Autodesk Fusion 360 part; units mm, degrees
(part 2 of 3)
sketch "dflg_DummyKey_Top_172" plane through (0, 0, -8.8) normal (0, 0, 1) x (1, 0, 0)
  line L0 (171.4, 78.4) -> (184.6, 78.4)
  line L1 (184.6, 78.4) -> (184.6, 91.6)
  line L2 (184.6, 91.6) -> (171.4, 91.6)
  line L3 (171.4, 91.6) -> (171.4, 78.4)
extrude "Extrude556" add sketch "dflg_DummyKey_Top_172" against normal blind 1.2 bodies 12
sketch "dflg_DummyKey_Top_142" plane through (0, 0, -8.8) normal (0, 0, 1) x (1, 0, 0)
  line L0 (141.4, 78.4) -> (154.6, 78.4)
  line L1 (154.6, 78.4) -> (154.6, 91.6)
  line L2 (154.6, 91.6) -> (141.4, 91.6)
  line L3 (141.4, 91.6) -> (141.4, 78.4)
extrude "Extrude557" add sketch "dflg_DummyKey_Top_142" against normal blind 1.2 bodies 13
sketch "dflg_DummyKey_Top_187" plane through (0, 0, -8.8) normal (0, 0, 1) x (1, 0, 0)
  line L0 (186.4, 78.4) -> (199.6, 78.4)
  line L1 (199.6, 78.4) -> (199.6, 91.6)
  line L2 (199.6, 91.6) -> (186.4, 91.6)
  line L3 (186.4, 91.6) -> (186.4, 78.4)
extrude "Extrude558" add sketch "dflg_DummyKey_Top_187" against normal blind 1.2 bodies 14
sketch "dflg_DummyKey_Top_202" plane through (0, 0, -8.8) normal (0, 0, 1) x (1, 0, 0)
  line L0 (201.4, 78.4) -> (214.6, 78.4)
  line L1 (214.6, 78.4) -> (214.6, 91.6)
  line L2 (214.6, 91.6) -> (201.4, 91.6)
  line L3 (201.4, 91.6) -> (201.4, 78.4)
extrude "Extrude559" add sketch "dflg_DummyKey_Top_202" against normal blind 1.2 bodies 15
sketch "dflg_DummyKey_Bot_157" plane through (0, 0, -8.8) normal (0, 0, 1) x (1, 0, 0)
  line L0 (156.4, 63.4) -> (169.6, 63.4)
  line L1 (169.6, 63.4) -> (169.6, 76.6)
  line L2 (169.6, 76.6) -> (156.4, 76.6)
  line L3 (156.4, 76.6) -> (156.4, 63.4)
extrude "Extrude560" add sketch "dflg_DummyKey_Bot_157" against normal blind 1.2 bodies 16
sketch "dflg_DummyKey_Bot_187" plane through (0, 0, -8.8) normal (0, 0, 1) x (1, 0, 0)
  line L0 (186.4, 63.4) -> (199.6, 63.4)
  line L1 (199.6, 63.4) -> (199.6, 76.6)
  line L2 (199.6, 76.6) -> (186.4, 76.6)
  line L3 (186.4, 76.6) -> (186.4, 63.4)
extrude "Extrude561" add sketch "dflg_DummyKey_Bot_187" against normal blind 1.2 bodies 17
sketch "dflg_DummyKey_Bot_142" plane through (0, 0, -8.8) normal (0, 0, 1) x (1, 0, 0)
  line L0 (141.4, 63.4) -> (154.6, 63.4)
  line L1 (154.6, 63.4) -> (154.6, 76.6)
  line L2 (154.6, 76.6) -> (141.4, 76.6)
  line L3 (141.4, 76.6) -> (141.4, 63.4)
extrude "Extrude562" add sketch "dflg_DummyKey_Bot_142" against normal blind 1.2 bodies 18
sketch "dflg_DummyKey_Bot_172" plane through (0, 0, -8.8) normal (0, 0, 1) x (1, 0, 0)
  line L0 (171.4, 63.4) -> (184.6, 63.4)
  line L1 (184.6, 63.4) -> (184.6, 76.6)
  line L2 (184.6, 76.6) -> (171.4, 76.6)
  line L3 (171.4, 76.6) -> (171.4, 63.4)
extrude "Extrude563" add sketch "dflg_DummyKey_Bot_172" against normal blind 1.2 bodies 19
sketch "dflg_DummyKey_Bot_202" plane through (0, 0, -8.8) normal (0, 0, 1) x (1, 0, 0)
  line L0 (201.4, 63.4) -> (214.6, 63.4)
  line L1 (214.6, 63.4) -> (214.6, 76.6)
  line L2 (214.6, 76.6) -> (201.4, 76.6)
  line L3 (201.4, 76.6) -> (201.4, 63.4)
extrude "Extrude564" add sketch "dflg_DummyKey_Bot_202" against normal blind 1.2 bodies 20
sketch "dflg_DummyBtn_Small_142" plane through (0, 0, -8.8) normal (0, 0, 1) x (1, 0, 0)
  line L0 (141.4, 39.4) -> (153.6, 39.4)
  line L1 (153.6, 39.4) -> (153.6, 51.6)
  line L2 (153.6, 51.6) -> (141.4, 51.6)
  line L3 (141.4, 51.6) -> (141.4, 39.4)
extrude "Extrude565" add sketch "dflg_DummyBtn_Small_142" against normal blind 1.2 bodies 21
sketch "dflg_DummyBtn_Small_155" plane through (0, 0, -8.8) normal (0, 0, 1) x (1, 0, 0)
  line L0 (154.4, 39.4) -> (166.6, 39.4)
  line L1 (166.6, 39.4) -> (166.6, 51.6)
  line L2 (166.6, 51.6) -> (154.4, 51.6)
  line L3 (154.4, 51.6) -> (154.4, 39.4)
extrude "Extrude566" add sketch "dflg_DummyBtn_Small_155" against normal blind 1.2 bodies 22
sketch "dflg_DummyBtn_Wide_139" plane through (0, 0, -8.8) normal (0, 0, 1) x (1, 0, 0)
  line L0 (138.4, 9.4) -> (165.6, 9.4)
  line L1 (165.6, 9.4) -> (165.6, 21.6)
  line L2 (165.6, 21.6) -> (138.4, 21.6)
  line L3 (138.4, 21.6) -> (138.4, 9.4)
extrude "Extrude568" add sketch "dflg_DummyBtn_Wide_139" against normal blind 1.2 bodies 23
sketch "dflg_DummyBtn_Wide_190" plane through (0, 0, -8.8) normal (0, 0, 1) x (1, 0, 0)
  line L0 (189.4, 9.4) -> (216.6, 9.4)
  line L1 (216.6, 9.4) -> (216.6, 21.6)
  line L2 (216.6, 21.6) -> (189.4, 21.6)
  line L3 (189.4, 21.6) -> (189.4, 9.4)
extrude "Extrude569" add sketch "dflg_DummyBtn_Wide_190" against normal blind 1.2 bodies 24
sketch "dflg_DummyPill_186" plane through (0, 0, -8.8) normal (0, 0, 1) x (1, 0, 0)
  line L0 (185.4, 45.4) -> (199.6, 45.4)
  line L1 (199.6, 45.4) -> (199.6, 50.6)
  line L2 (199.6, 50.6) -> (185.4, 50.6)
  line L3 (185.4, 50.6) -> (185.4, 45.4)
extrude "Extrude570" add sketch "dflg_DummyPill_186" against normal blind 1.2 bodies 25
sketch "dflg_DummyPill_202" plane through (0, 0, -8.8) normal (0, 0, 1) x (1, 0, 0)
  line L0 (201.4, 45.4) -> (215.6, 45.4)
  line L1 (215.6, 45.4) -> (215.6, 50.6)
  line L2 (215.6, 50.6) -> (201.4, 50.6)
  line L3 (201.4, 50.6) -> (201.4, 45.4)
extrude "Extrude571" add sketch "dflg_DummyPill_202" against normal blind 1.2 bodies 26
extrude "Extrude578" add 1 faces at (104.2, 86.8333, -11) along direction (0, 0, 1) blind 7 on bodies 1 bodies 1
extrude "Extrude579" add 1 faces at (102, 86.8333, -4.8) along direction (1, 0, 0) blind 1 on bodies 1 bodies 1
extrude "Extrude580" add 1 faces at (120.7617, 93, -3.3333) along direction (0, -1, 0) blind 16 on bodies 4 bodies 4
extrude "Extrude581" add 1 faces at (126.6667, 83.1667, -11) along direction (0, 0, 1) blind 8 on bodies 4 bodies 4
fillet "Fillet36" radius 2 1 edges at (130, 85, -3) on bodies 4
ref_plane "WorkPlane54" through (0, 0, -3.7) normal (0, 0, 1) x (1, 0, 0)
ref_plane "WorkPlane55" through (0, 0, -6.6) normal (0, 0, 1) x (1, 0, 0)
ref_plane "WorkPlane56" through (0, 0, -3.7) normal (0, 0, 1) x (1, 0, 0)
ref_plane "WorkPlane57" through (0, 0, -6.6) normal (0, 0, 1) x (1, 0, 0)
ref_plane "WorkPlane58" through (0, 0, -3.7) normal (0, 0, 1) x (1, 0, 0)
ref_plane "WorkPlane59" through (0, 0, -6.6) normal (0, 0, 1) x (1, 0, 0)
ref_plane "WorkPlane60" through (0, 0, -3.7) normal (0, 0, 1) x (1, 0, 0)
ref_plane "WorkPlane61" through (0, 0, -6.6) normal (0, 0, 1) x (1, 0, 0)
ref_plane "WorkPlane62" through (0, 0, -3.7) normal (0, 0, 1) x (1, 0, 0)
ref_plane "WorkPlane63" through (0, 0, -6.6) normal (0, 0, 1) x (1, 0, 0)
ref_plane "WorkPlane64" through (0, 0, -3.7) normal (0, 0, 1) x (1, 0, 0)
ref_plane "WorkPlane65" through (0, 0, -6.4) normal (0, 0, 1) x (1, 0, 0)
extrude "Extrude645" cut 1 faces at (63.1792, 74.7218, -20.4) along direction (0, 0, 1) blind 14 on bodies 1 bodies 1
extrude "Extrude646" cut 1 faces at (59.609, 74.3228, -15.9) along direction (0, 0, 1) blind 9.5 on bodies 1 bodies 1
extrude "Extrude647" add 1 faces at (96.6851, 105.8013, -16.4) along direction (0, 0, -1) blind 8 on bodies 1 bodies 1
extrude "Extrude648" add 1 faces at (14.3667, 106, -16.4) along direction (0, 0, -1) blind 8 on bodies 1 bodies 1
extrude "Extrude649" add 1 faces at (83, 113.2, -6.1333) along direction (-1, 0, 0) blind 3 on bodies 1 bodies 1
extrude "Extrude650" cut 1 faces at (14.3667, 106, -24.4) along direction (0, 0, 1) blind 3 on bodies 1 bodies 1
extrude "Extrude651" cut 1 faces at (96.6851, 105.8013, -24.4) along direction (0, 0, 1) blind 3 on bodies 1 bodies 1
extrude "Extrude652" add 1 faces at (96.6851, 105.8013, -21.4) along direction (0, 0, -1) blind 0.5 on bodies 1 bodies 1
extrude "Extrude653" add 1 faces at (14.3667, 106, -21.4) along direction (0, 0, -1) blind 0.5 on bodies 1 bodies 1
move_face "MoveFace1" by (-5, 0, 0) 1 faces at (86.3, 115.1, -5.6) on bodies 1
extrude "Extrude654" add 1 faces at (88.5, 81.5, -5.8667) along direction (-1, 0, 0) blind 23 on bodies 1 bodies 1
extrude "Extrude655" add 1 faces at (88.5, 78.6833, -5.8667) along direction (-1, 0, 0) blind 23 on bodies 1 bodies 1
extrude "Extrude656" cut 1 faces at (24.7, 98.8, -6.1333) along direction (-1, 0, 0) blind 1 on bodies 1 bodies 1
extrude "Extrude657" add 1 faces at (80, 113.2, -6.1333) along direction (-1, 0, 0) blind 2 on bodies 1 bodies 1
extrude "Extrude658" add 1 faces at (65.5, 75.3, -5.3333) along direction (1, 0, 0) blind 9 on bodies 1 bodies 1
extrude "Extrude659" add 4 faces at (65.5, 73, -4.8) (65.5, 70, -4.8) (65.5, 67, -4.8) (65.5, 64, -4.8) along direction (1, 0, 0) blind 9 on bodies 1 bodies 1
extrude "Extrude660" add 1 faces at (77.5, 75.9, -4.5333) along direction (0, -1, 0) blind 1 on bodies 1 bodies 1
extrude "Extrude661" add 1 faces at (77.5, 76, -5.6) along direction (0, 0, -1) blind 0.7 on bodies 1 bodies 1
extrude "Extrude662" add 1 faces at (77.5, 76, -6.3) along direction (0, 0, -1) blind 0.1 on bodies 1 bodies 1
extrude "Extrude663" cut 1 faces at (10.1851, 75.8013, -20.4) along direction (0, 0, 1) blind 4.5 on bodies 1 bodies 1
extrude "Extrude664" cut 1 faces at (4.8353, 75.2763, -15.9) along direction (0, 0, 1) blind 9.5 on bodies 1 bodies 1
extrude "Extrude665" cut 1 faces at (94.1792, 53.7218, -20.4) along direction (0, 0, 1) blind 4.5 on bodies 1 bodies 1
extrude "Extrude666" cut 1 faces at (88.7042, 55.1056, -15.9) along direction (0, 0, 1) blind 9.5 on bodies 1 bodies 1
extrude "Extrude667" cut 1 faces at (51.1892, 20.6651, -20.4) along direction (0, 0, 1) blind 4.5 on bodies 1 bodies 1
extrude "Extrude668" cut 1 faces at (48.3181, 21.1557, -15.9) along direction (0, 0, 1) blind 9.5 on bodies 1 bodies 1
extrude "Extrude669" cut 1 faces at (12.1792, 24.7218, -20.4) along direction (0, 0, 1) blind 4.5 on bodies 1 bodies 1
extrude "Extrude670" cut 1 faces at (8.7033, 26.2999, -15.9) along direction (0, 0, 1) blind 9.5 on bodies 1 bodies 1
ref_plane "WorkPlane66" through (52.5, 80.0825, -6.4) normal (0, 0, -1) x (-1, 0, 0)
sketch "Sketch596" plane through (0, 0, -6.4) normal (0, 0, -1) x (-1, 0, 0)
  line L0 (-2.4, 78.2245) -> (-8.4, 78.2245)
  line L1 (-8.4, 78.2245) -> (-8.4, 16.2245)
  line L2 (-8.4, 16.2245) -> (-2.4, 16.2245)
  line L3 (-2.4, 16.2245) -> (-2.4, 78.2245)
  line L4 (-2.4, 6) -> (-2.4, 138.2533)
  dimension "d1957" = 6
  dimension "d1958" = 62
  constraint horizontal L0
  constraint vertical L1
  constraint horizontal L2
  constraint vertical L3
  constraint coincident L0.start L4
  measures "d1957" distance of L0.start L0.end
  measures "d1958" distance of L0.start L2.end
extrude "Extrude671" add sketch "Sketch596" along normal blind 3 bodies 1
extrude "Extrude672" cut 1 faces at (4.4, 36.8912, -9.4) along direction (0, 0, 1) blind 1 on bodies 1 bodies 1
sketch "Sketch597" plane through (0, 0, -8.4) normal (0, 0, -1) x (1, 0, 0)
  line L0 (8.4, -16.2245) -> (2.4, -16.2245)
  line L1 (2.4, -16.2245) -> (2.4, -78.2245)
  line L2 (2.4, -78.2245) -> (8.4, -78.2245)
  line L3 (8.4, -78.2245) -> (8.4, -16.2245)
  circle A0 centre (5, -73) radius 1.6
  circle A1 centre (5, -51) radius 1.6
  circle A2 centre (5, -29) radius 1.6
  circle A3 centre (68, -70) radius 1.6
  circle A4 centre (53, -29) radius 1.6
  circle A5 centre (69, -73) radius 1.6
  circle A6 centre (69, -73) radius 1.6
  circle A7 centre (69.5, -72.5) radius 1.6
  dimension "d1963" = 3.2
  dimension "d1966" = 0
  dimension "d1967" = 44
  dimension "d1980" = 3.2
  dimension "d2000" = 3.2
  dimension "d2003" = 3.2
  dimension "d2016" = 3.2
  constraint concentric A5 A6
  measures "d1963" diameter of A0
  measures "d1980" diameter of A3
  measures "d2000" diameter of A5
  measures "d2003" diameter of A6
  measures "d2016" diameter of A7
extrude "Extrude673" add sketch "Sketch597" along normal blind 1 contours L0 L1 L2 L3 bodies 1
extrude "Extrude674" cut 3 faces at (4.8052, 72.5035, -8.4) (5.391, 51.3628, -8.4) (4.7333, 28.5381, -8.4) along direction (0, 0, 1) blind 2.5 on bodies 1 bodies 1
extrude "Extrude675" add 4 faces at (74.5, 73, -4.8) (74.5, 70, -4.8) (74.5, 67, -4.8) (74.5, 64, -4.8) along direction (1, 0, 0) blind 5 on bodies 1 bodies 1
extrude "Extrude676" cut 4 faces at (83.5, 63.5, -4.8) (83.5, 66.5, -4.8) (83.5, 69.5, -4.8) (83.5, 72.5, -4.8) along direction (1, 0, 0) blind 11 on bodies 1 bodies 1
sketch "Sketch598" plane through (0, 0, -6.4) normal (0, 0, -1) x (1, 0, 0)
  line L0 (8.4, -78.2245) -> (2.4, -78.2245)
  line L1 (2.4, -78.2245) -> (2.4, -138.2533)
  arc A0 (53.3792, -143.3184) -> (2.4, -138.2533) centre (11.7114, -303.6168) ccw
  arc A1 (102.6, -157.7649) -> (53.3792, -143.3184) centre (-358, -1636) ccw
  line L2 (102.6, -157.7649) -> (102.6, -6)
  arc A2 (102.6, -6) -> (99, -2.4) centre (99, -6) ccw
  line L3 (99, -2.4) -> (6, -2.4)
  arc A3 (6, -2.4) -> (2.4, -6) centre (6, -6) ccw
  line L4 (2.4, -6) -> (2.4, -16.2245)
  line L5 (2.4, -16.2245) -> (8.4, -16.2245)
  line L6 (8.4, -16.2245) -> (8.4, -78.2245)
  circle A4 centre (40, -69) radius 7.2
  circle A5 centre (30, -32.5) radius 7.2
  circle A6 centre (93.5, -106) radius 4
  line L7 (76.65, -139.05) -> (88.65, -139.05)
  line L8 (88.65, -139.05) -> (88.65, -142.05)
  line L9 (88.65, -142.05) -> (76.65, -142.05)
  line L10 (76.65, -142.05) -> (76.65, -139.05)
  circle A7 centre (93, -11.5) radius 4.2
  circle A8 centre (11.5, -11.5) radius 4.2
  line L11 (59, -25.8) -> (71.3, -25.8)
  line L12 (71.3, -25.8) -> (71.3, -13.5)
  line L13 (71.3, -13.5) -> (83.7, -13.5)
  line L14 (83.7, -13.5) -> (83.7, -25.8)
  line L15 (83.7, -25.8) -> (96, -25.8)
  line L16 (96, -25.8) -> (96, -38.2)
  line L17 (96, -38.2) -> (83.7, -38.2)
  line L18 (83.7, -38.2) -> (83.7, -50.5)
  line L19 (83.7, -50.5) -> (71.3, -50.5)
  line L20 (71.3, -50.5) -> (71.3, -38.2)
  line L21 (71.3, -38.2) -> (59, -38.2)
  line L22 (59, -38.2) -> (59, -25.8)
  line L23 (61.8432, -78.55) -> (88.65, -78.55)
  line L24 (88.65, -78.55) -> (88.65, -130.45)
  line L25 (88.65, -130.45) -> (85.65, -130.45)
  line L26 (85.65, -130.45) -> (85.65, -81.55)
  line L27 (85.65, -81.55) -> (18.95, -81.55)
  line L28 (18.95, -81.55) -> (18.95, -130.45)
  line L29 (18.95, -130.45) -> (15.95, -130.45)
  line L30 (15.95, -130.45) -> (15.95, -78.55)
  line L31 (15.95, -78.55) -> (58.1568, -78.55)
  arc A9 (58.1568, -78.55) -> (61.8432, -78.55) centre (60, -75) ccw
  line L32 (19.5567, -75.9) -> (15.4433, -75.9)
  arc A10 (19.5567, -75.9) -> (15.4433, -75.9) centre (17.5, -69) ccw
  line L33 (49.5, -54) -> (64.5, -54)
  line L34 (64.5, -54) -> (64.5, -58)
  line L35 (64.5, -58) -> (49.5, -58)
  line L36 (49.5, -58) -> (49.5, -54)
  line L37 (30.5, -54) -> (45.5, -54)
  line L38 (45.5, -54) -> (45.5, -58)
  line L39 (45.5, -58) -> (30.5, -58)
  line L40 (30.5, -58) -> (30.5, -54)
  circle A11 centre (93, -80) radius 4.2
  circle A12 centre (11.5, -85) radius 4.2
  circle A13 centre (93, -120) radius 4.2
  circle A14 centre (11.5, -106) radius 4
  line L41 (78, -127.6) -> (23.7, -127.6)
  line L42 (23.7, -127.6) -> (23.7, -84.4)
  line L43 (23.7, -84.4) -> (78, -84.4)
  line L44 (78, -84.4) -> (78, -127.6)
  line L45 (94.5, -73.5) -> (79.5, -73.5)
  line L46 (79.5, -73.5) -> (79.5, -72)
  line L47 (79.5, -72) -> (94.5, -72)
  line L48 (94.5, -72) -> (94.5, -73.5)
  line L49 (94.5, -67.5) -> (79.5, -67.5)
  line L50 (79.5, -67.5) -> (79.5, -66)
  line L51 (79.5, -66) -> (94.5, -66)
  line L52 (94.5, -66) -> (94.5, -67.5)
  line L53 (94.5, -64.5) -> (79.5, -64.5)
  line L54 (79.5, -64.5) -> (79.5, -63)
  line L55 (79.5, -63) -> (94.5, -63)
  line L56 (94.5, -63) -> (94.5, -64.5)
  line L57 (94.5, -70.5) -> (79.5, -70.5)
  line L58 (79.5, -70.5) -> (79.5, -69)
  line L59 (79.5, -69) -> (94.5, -69)
  line L60 (94.5, -69) -> (94.5, -70.5)
  line L61 (83.2556, -76.4857) -> (65.2556, -76.4857)
  line L62 (65.2556, -76.4857) -> (65.2556, -52.4857)
  line L63 (65.2556, -52.4857) -> (83.2556, -52.4857)
  line L64 (83.2556, -52.4857) -> (83.2556, -76.4857)
  line L65 (58, -45) -> (49, -45)
  line L66 (49, -45) -> (49, -17)
  line L67 (49, -17) -> (58, -17)
  line L68 (58, -17) -> (58, -45)
  dimension "d1976" = 24
  dimension "d1977" = 18
  constraint horizontal L61
  constraint vertical L62
  constraint horizontal L63
  constraint vertical L64
  constraint horizontal L65
  constraint vertical L66
  constraint horizontal L67
  constraint vertical L68
  measures "d1976" distance of L61.start L63.end
  measures "d1977" distance of L61.start L61.end
extrude "Extrude678" add sketch "Sketch598" along normal blind 3 contours L65 L66 L67 L68 bodies 1
extrude "Extrude679" cut sketch "Sketch597" against normal blind 3.5 contours A3 A7 | A3 A5 A6 A7 | A3 A5 A6 picked at (68.8187, -71.1587) bodies 1
sketch "Sketch599" plane through (0, 0, -9.4) normal (0, 0, -1) x (1, 0, 0)
  line L0 (58, -17) -> (49, -17)
  line L1 (49, -17) -> (49, -45)
  line L2 (49, -45) -> (58, -45)
  line L3 (58, -45) -> (58, -17)
  circle A0 centre (53, -29) radius 1.6
  circle A1 centre (54, -30) radius 1.6
  dimension "d1986" = 3.2
  dimension "d2007" = 3.2
  measures "d1986" diameter of A0
  measures "d2007" diameter of A1
extrude "Extrude680" cut sketch "Sketch599" against normal blind 3.5 contours A0 A1 | A0 A1 picked at (53.3119, -29.2702) picked at (52.5374, -28.5374) bodies 1
extrude "Extrude681" add 4 faces at (79.5, 73, -4.8) (79.5, 70, -4.8) (79.5, 67, -4.8) (79.5, 64, -4.8) along direction (1, 0, 0) blind 6.5 on bodies 1 bodies 1
extrude "Extrude682" cut 4 faces at (94.5, 72.5, -4.8) (94.5, 69.5, -4.8) (94.5, 66.5, -4.8) (94.5, 63.5, -4.8) along direction (1, 0, 0) blind 5 on bodies 1 bodies 1
extrude "Extrude683" add sketch "Sketch598" along normal blind 3 contours L45 L46 L47 L49 L50 L51 L53 L54 L55 L57 L58 L59 L61 L62 L63 L64 | L45 L46 L47 L64 | L57 L58 L59 L64 | L49 L50 L51 L64 | L53 L54 L55 L64 bodies 1
sketch "Sketch600" plane through (0, 0, -9.4) normal (0, 0, -1) x (1, 0, 0)
  line L0 (83.2556, -52.4857) -> (65.2556, -52.4857)
  line L1 (65.2556, -52.4857) -> (65.2556, -76.4857)
  line L2 (65.2556, -76.4857) -> (83.2556, -76.4857)
  line L3 (83.2556, -76.4857) -> (83.2556, -52.4857)
  circle A0 centre (77, -59) radius 1.6
  dimension "d2028" = 3.2
  measures "d2028" diameter of A0
extrude "Extrude685" add sketch "Sketch597" along normal blind 1 contours A3 A7 | A3 A5 A6 A7 picked at (68.8187, -71.1587) bodies 1
extrude "Extrude687" add sketch "Sketch599" along normal blind 1 separate body contours A0 A1 | A0 A1 picked at (53.3119, -29.2702) picked at (52.5374, -28.5374) makes body 27
extrude "Extrude688" cut 1 faces at (53.4404, 28.6598, -10.4) along direction (0, 0, 1) blind 1 on bodies 27 bodies 27
extrude "Extrude689" add sketch "Sketch597" along normal blind 1 contours A4 bodies 1 27
extrude "Extrude690" cut sketch "Sketch599" against normal blind 3.5 contours A0 A1 | A0 A1 picked at (53.3119, -29.2702) picked at (54.988, -30.5494) bodies 1
extrude "Extrude691" add sketch "Sketch597" along normal blind 1 separate body contours A5 A6 A7 makes body 28
sketch "Sketch602" plane through (0, 0, -9.4) normal (0, 0, -1) x (1, 0, 0)
  circle A0 centre (69.5, -72.5) radius 1.6
  dimension "d2019" = 3.2
  measures "d2019" diameter of A0
extrude "Extrude692" cut sketch "Sketch602" against normal blind 3.5 bodies 1
extrude "Extrude693" add sketch "Sketch600" against normal blind 5 contours L0 L1 L2 L3 | A0 bodies 1 28
extrude "Extrude694" cut sketch "Sketch602" against normal blind 3.5 bodies 1
sketch "Sketch603" plane through (0, 0, -6.4) normal (0, 0, -1) x (1, 0, 0)
sketch "Sketch604" plane through (0, 0, -6.4) normal (0, 0, -1) x (1, 0, 0)
  line L0 (49, -17) -> (49, -6)
  line L1 (49, -6) -> (69, -6)
  line L2 (69, -6) -> (69, -17)
  line L3 (69, -17) -> (49, -17)
  line L4 (58, -24) -> (68, -24)
  line L5 (68, -24) -> (68, -17)
  line L6 (68, -17) -> (58, -17)
  line L7 (58, -17) -> (58, -24)
  line L8 (58, -40) -> (69, -40)
  line L9 (69, -40) -> (69, -51)
  line L10 (69, -51) -> (58, -51)
  line L11 (58, -51) -> (58, -40)
  line L12 (86, -16) -> (86, -25)
  line L13 (86, -25) -> (101.3332, -25)
  line L14 (101.3332, -25) -> (101.3332, -16)
  line L15 (101.3332, -16) -> (86, -16)
  line L16 (97, -25) -> (97, -57)
  line L17 (97, -57) -> (102, -57)
  line L18 (102, -57) -> (102, -25)
  line L19 (102, -25) -> (97, -25)
  line L20 (97, -41) -> (86, -41)
  line L21 (86, -41) -> (86, -57)
  line L22 (86, -57) -> (97, -57)
  line L23 (97, -57) -> (97, -41)
  constraint perpendicular L0 L1
  constraint parallel L0 L2
  constraint parallel L1 L3
  constraint vertical L0
  constraint perpendicular L4 L5
  constraint parallel L4 L6
  constraint parallel L5 L7
  constraint perpendicular L2 L4
  constraint perpendicular L8 L9
  constraint parallel L8 L10
  constraint parallel L9 L11
  constraint horizontal L8
  constraint perpendicular L12 L13
  constraint parallel L12 L14
  constraint parallel L13 L15
  constraint perpendicular L10 L12
  constraint perpendicular L16 L17
  constraint parallel L16 L18
  constraint parallel L17 L19
  constraint perpendicular L13 L16
  constraint coincident L13 L16.start
  constraint perpendicular L20 L21
  constraint parallel L20 L22
  constraint parallel L21 L23
  constraint perpendicular L16 L20
  constraint midpoint L16 L20.start
extrude "Extrude695" add sketch "Sketch604" along normal blind 3 bodies 1
sketch "Sketch605" plane through (0, 0, -9.4) normal (0, 0, -1) x (1, 0, 0)
  circle A0 centre (54, -30) radius 1.6
  line L0 (49, -6) -> (49, -45)
  line L1 (49, -45) -> (58, -45)
  line L2 (58, -45) -> (58, -51)
  line L3 (58, -51) -> (69, -51)
  line L4 (69, -51) -> (69, -40)
  line L5 (69, -40) -> (58, -40)
  line L6 (58, -40) -> (58, -24)
  line L7 (58, -24) -> (68, -24)
  line L8 (68, -24) -> (68, -17)
  line L9 (68, -17) -> (69, -17)
  line L10 (69, -17) -> (69, -6)
  line L11 (69, -6) -> (49, -6)
  circle A1 centre (63, -11) radius 1.6
  dimension "d2029" = 3.2
  measures "d2029" diameter of A1
sketch "Sketch606" plane through (0, 0, -9.4) normal (0, 0, -1) x (1, 0, 0)
  line L0 (86, -57) -> (102, -57)
  line L1 (102, -57) -> (102, -25)
  line L2 (102, -25) -> (101.3332, -25)
  line L3 (101.3332, -25) -> (101.3332, -16)
  line L4 (101.3332, -16) -> (86, -16)
  line L5 (86, -16) -> (86, -25)
  line L6 (86, -25) -> (97, -25)
  line L7 (97, -25) -> (97, -41)
  line L8 (97, -41) -> (86, -41)
  line L9 (86, -41) -> (86, -57)
  circle A0 centre (95, -47) radius 1.6
  circle A1 centre (92, -21) radius 1.6
  dimension "d2030" = 3.2
  dimension "d2031" = 3.2
  measures "d2030" diameter of A0
  measures "d2031" diameter of A1
extrude "Extrude696" cut sketch "Sketch606" against normal blind 3.5 contours A0 | A1 bodies 1
extrude "Extrude697" cut sketch "Sketch605" against normal blind 3.5 contours A1 bodies 1
extrude "Extrude698" cut sketch "Sketch600" against normal blind 3.5 contours A0 bodies 1
sketch "Sketch607" plane through (0, 0, -9.4) normal (0, 0, -1) x (1, 0, 0)
  circle A0 centre (63, -11) radius 1.6
  circle A1 centre (54, -30) radius 1.6
  line L0 (49, -6) -> (49, -45)
  line L1 (49, -45) -> (58, -45)
  line L2 (58, -45) -> (58, -51)
  line L3 (58, -51) -> (69, -51)
  line L4 (69, -51) -> (69, -40)
  line L5 (69, -40) -> (58, -40)
  line L6 (58, -40) -> (58, -24)
  line L7 (58, -24) -> (68, -24)
  line L8 (68, -24) -> (68, -17)
  line L9 (68, -17) -> (69, -17)
  line L10 (69, -17) -> (69, -6)
  line L11 (69, -6) -> (49, -6)
  circle A2 centre (65, -45) radius 1.75
  dimension "d2038" = 3.5
  measures "d2038" diameter of A2
extrude "Extrude699" cut sketch "Sketch607" against normal blind 3.5 contours A2 bodies 1
extrude "Extrude677" add sketch "Sketch598" along normal blind 3 contours L45 L46 L47 L49 L50 L51 L53 L54 L55 L57 L58 L59 L61 L62 L63 L64 | L45 L46 L47 L64 | L57 L58 L59 L64 | L49 L50 L51 L64 | L53 L54 L55 L64 bodies 1
ref_plane "WorkPlane67" through (0, 155, 0) normal (0, 1, 0) x (0, 0, 1)
sketch "Sketch614" plane through (0, 0, -8) normal (0, 0, -1) x (1, 0, 0)
  line L0 (15.95, -142.05) -> (15.95, -141.849)
  arc A0 (15.95, -141.849) -> (14.1534, -167.6) centre (19, -155) ccw
  line L1 (14.1534, -167.6) -> (23.8466, -167.6)
  arc A1 (23.8466, -167.6) -> (22.8141, -142.05) centre (19, -155) ccw
  line L2 (22.8141, -142.05) -> (15.95, -142.05)
  circle A2 centre (11.5, -156) radius 4.2
sketch "Sketch615" plane through (0, 0, 5.8) normal (0, 0, 1) x (-1, 0, 0)
  circle A0 centre (-19, -155) radius 13.5
  circle A1 centre (-19, -155) radius 1.5
  dimension "d2062" = 3
  constraint concentric A0 A1
  measures "d2062" diameter of A1
extrude "Extrude703" cut sketch "Sketch615" against normal blind 30 contours A1 bodies 1
extrude "Extrude704" cut sketch "Sketch602" against normal blind 3.5 bodies 1
sketch "Sketch616" plane through (0, 0, -9.4) normal (0, 0, -1) x (1, 0, 0)
  circle A0 centre (69.5, -72.5) radius 1.6
  line L0 (83.2556, -52.4857) -> (65.2556, -52.4857)
  line L1 (65.2556, -52.4857) -> (65.2556, -76.4857)
  line L2 (65.2556, -76.4857) -> (83.2556, -76.4857)
  line L3 (83.2556, -76.4857) -> (83.2556, -52.4857)
  circle A1 centre (77, -59) radius 1.6
  dimension "d2067" = 3.2
  measures "d2067" diameter of A1
extrude "Extrude705" cut sketch "Sketch616" against normal blind 3.5 contours A1 bodies 1
extrude "Extrude706" add sketch "Sketch599" against normal blind 3.5 contours A0 A1 picked at (52.5374, -28.5374) bodies 1
extrude "Extrude707" cut 1 faces at (40.5, 58, -4.8) along direction (0, 1, 0) blind 0.5 on bodies 1 bodies 1
extrude "Extrude708" cut 1 faces at (59.5, 58, -4.8) along direction (0, 1, 0) blind 0.5 on bodies 1 bodies 1
extrude "Extrude709" cut 1 faces at (54.5, 54, -4.8) along direction (0, -1, 0) blind 0.5 on bodies 1 bodies 1
extrude "Extrude710" cut 1 faces at (35.5, 54, -4.8) along direction (0, -1, 0) blind 0.5 on bodies 1 bodies 1
sketch "Sketch617" plane through (0, 0, -8) normal (0, 0, -1) x (1, 0, 0)
  circle A0 centre (19, -155) radius 1.5
  dimension "d2080" = 3
  measures "d2080" diameter of A0
extrude "Extrude711" add sketch "Sketch617" against normal blind 13.4 bodies 1
sketch "Sketch618" plane through (0, 0, 5.8) normal (0, 0, 1) x (-1, 0, 0)
  circle A0 centre (-19, -155) radius 1.5
  circle A1 centre (-19, -155) radius 13.5
  line L0 (-11.5, -150) -> (-26.5, -150)
  line L1 (-26.5, -150) -> (-26.5, -160)
  line L2 (-26.5, -160) -> (-11.5, -160)
  line L3 (-11.5, -160) -> (-11.5, -150)
  line L4 (-11.5, -150) -> (-26.5, -160) construction
  line L5 (-26.5, -150) -> (-11.5, -160) construction
  point P0 (-19, -155)
  dimension "d2083" = 15
  dimension "d2084" = 10
  constraint horizontal L0
  constraint perpendicular L0 L1
  constraint parallel L0 L2
  constraint parallel L1 L3
  constraint coincident L4 P0
  constraint coincident L5 P0
  constraint coincident P0 A0.centre
  measures "d2083" distance of L1.end L2.end
  measures "d2084" distance of L0.end L1.end
extrude "Extrude712" cut sketch "Sketch618" against normal blind 0.5 contours L0 L1 L2 L3 bodies 1
extrude "Extrude713" cut 1 faces at (19.25, 155.433, 5.4) along direction (0, 0, -1) blind 0.2 on bodies 1 bodies 1
extrude "Extrude714" add 1 faces at (19.25, 155.433, 5.2) along direction (0, 0, 1) blind 0.1 on bodies 1 bodies 1
sketch "Sketch619" plane through (0, 0, 5.8) normal (0, 0, 1) x (-1, 0, 0)
  line L0 (-26.5, -150) -> (-11.5, -150)
  line L1 (-11.5, -150) -> (-11.5, -160)
  line L2 (-11.5, -160) -> (-26.5, -160)
  line L3 (-26.5, -160) -> (-26.5, -150)
  circle A0 centre (-19, -155) radius 13.5
  line L4 (-27.5, -160) -> (-29, -160)
  line L5 (-29, -160) -> (-29, -150)
  line L6 (-29, -150) -> (-27.5, -150)
  line L7 (-27.5, -150) -> (-27.5, -160)
  constraint horizontal L4
  constraint vertical L5
  constraint horizontal L6
  constraint vertical L7
extrude "Extrude715" cut sketch "Sketch619" against normal blind 23 contours L4 L5 L6 L7 bodies 1
sketch "Sketch620" plane through (0, 0, -6.4) normal (0, 0, -1) x (1, 0, 0)
extrude "Extrude716" cut 1 faces at (54.5, 53.5, -4.8) along direction (0, -1, 0) blind 2.4 on bodies 1 bodies 1
extrude "Extrude717" cut 1 faces at (35.5, 53.5, -4.8) along direction (0, -1, 0) blind 2.4 on bodies 1 bodies 1
extrude "Extrude718" cut 4 faces at (61.891, 105.5419, -34) (9.891, 100.4419, -34) (9.891, 72.4419, -34) (60.591, 57.2419, -34) along direction (0, 0, -1) blind 6 on bodies 3 bodies 3
extrude "Extrude719" cut 1 faces at (40.5, 58.5, -4.8) along direction (0, 1, 0) blind 1.2 on bodies 1 bodies 1
extrude "Extrude720" cut 1 faces at (59.5, 58.5, -4.8) along direction (0, 1, 0) blind 1.2 on bodies 1 bodies 1
extrude "Extrude721" cut 1 faces at (8.1408, 84.1822, -44) along direction (0, 0, 1) blind 6 on bodies 1 bodies 1
extrude "Extrude722" cut 1 faces at (8.1408, 84.1822, -38) along direction (0, 0, 1) blind 0.5 on bodies 1 bodies 1
extrude "Extrude723" cut 1 faces at (8.3797, 84.2559, -37.5) along direction (0, 0, 1) blind 31 on bodies 1 bodies 1
extrude "Extrude724" cut 1 faces at (11.4689, 84.1151, -32.4) along direction (0, 0, 1) blind 26 on bodies 1 bodies 1
sketch "delboss_66_1007" plane through (0, 0, 0) normal (0, 0, 1) x (1, 0, 0)
  circle A0 centre (6.6, 100.7) radius 5.5
extrude "Extrude729" cut sketch "delboss_66_1007" along normal blind 4.02 from surface at -44.01 bodies 3
sketch "delboss_586_1058" plane through (0, 0, 0) normal (0, 0, 1) x (1, 0, 0)
  circle A0 centre (58.6, 105.8) radius 5.5
extrude "Extrude730" cut sketch "delboss_586_1058" along normal blind 4.02 from surface at -44.01 bodies 3
sketch "delboss_573_575" plane through (0, 0, 0) normal (0, 0, 1) x (1, 0, 0)
  circle A0 centre (57.3, 57.5) radius 5.5
extrude "Extrude731" cut sketch "delboss_573_575" along normal blind 4.02 from surface at -44.01 bodies 3
sketch "delboss_66_727" plane through (0, 0, 0) normal (0, 0, 1) x (1, 0, 0)
  circle A0 centre (6.6, 72.7) radius 5.5
extrude "Extrude732" cut sketch "delboss_66_727" along normal blind 4.02 from surface at -44.01 bodies 3
sketch "nboss_537_420" plane through (0, 0, 0) normal (0, 0, 1) x (1, 0, 0)
  circle A0 centre (53.7, 42) radius 4
extrude "Extrude733" add sketch "nboss_537_420" along normal blind 4 from surface at -44 bodies 3
sketch "nbore_537_420" plane through (0, 0, 0) normal (0, 0, 1) x (1, 0, 0)
  circle A0 centre (53.7, 42) radius 2
extrude "Extrude734" cut sketch "nbore_537_420" against normal blind 3 from surface at -40 bodies 3
sketch "nboss_588_940" plane through (0, 0, 0) normal (0, 0, 1) x (1, 0, 0)
  circle A0 centre (58.8, 94) radius 4
extrude "Extrude735" add sketch "nboss_588_940" along normal blind 4 from surface at -44 bodies 3
sketch "nbore_588_940" plane through (0, 0, 0) normal (0, 0, 1) x (1, 0, 0)
  circle A0 centre (58.8, 94) radius 2
extrude "Extrude736" cut sketch "nbore_588_940" against normal blind 3 from surface at -40 bodies 3
sketch "nboss_105_927" plane through (0, 0, 0) normal (0, 0, 1) x (1, 0, 0)
  circle A0 centre (10.5, 92.7) radius 4
extrude "Extrude737" add sketch "nboss_105_927" along normal blind 4 from surface at -44 bodies 3
sketch "nbore_105_927" plane through (0, 0, 0) normal (0, 0, 1) x (1, 0, 0)
  circle A0 centre (10.5, 92.7) radius 2
extrude "Extrude738" cut sketch "nbore_105_927" against normal blind 3 from surface at -40 bodies 3
sketch "nboss_257_420" plane through (0, 0, 0) normal (0, 0, 1) x (1, 0, 0)
  circle A0 centre (25.7, 42) radius 4
extrude "Extrude739" add sketch "nboss_257_420" along normal blind 4 from surface at -44 bodies 3
sketch "nbore_257_420" plane through (0, 0, 0) normal (0, 0, 1) x (1, 0, 0)
  circle A0 centre (25.7, 42) radius 2
extrude "Extrude740" cut sketch "nbore_257_420" against normal blind 3 from surface at -40 bodies 3
sketch "unoq_rot" plane through (0, 0, 0) normal (0, 0, 1) x (1, 0, 0)
  line L0 (8, 39.4) -> (61.3, 39.4)
  line L1 (61.3, 39.4) -> (61.3, 108)
  line L2 (61.3, 108) -> (8, 108)
  line L3 (8, 108) -> (8, 39.4)
extrude "Extrude741" add sketch "unoq_rot" along normal blind 9.6 from surface at -34 separate body makes body 29
sketch "usbc_rot" plane through (0, 0, 0) normal (0, 0, 1) x (1, 0, 0)
  line L0 (12, 108) -> (21, 108)
  line L1 (21, 108) -> (21, 111.4)
  line L2 (21, 111.4) -> (12, 111.4)
  line L3 (12, 111.4) -> (12, 108)
extrude "Extrude742" add sketch "usbc_rot" along normal blind 3.2 from surface at -34 separate body makes body 30
sketch "mount_base" plane through (0, 0, 0) normal (0, 0, 1) x (1, 0, 0)
  line L0 (127, 17) -> (201.6, 17)
  line L1 (201.6, 17) -> (201.6, 76.3)
  line L2 (201.6, 76.3) -> (127, 76.3)
  line L3 (127, 76.3) -> (127, 17)
extrude "Extrude743" add sketch "mount_base" along normal blind 3 separate body makes body 31
sketch "mstand_26_457" plane through (0, 0, 0) normal (0, 0, 1) x (1, 0, 0)
  circle A0 centre (132.6, 65.7) radius 3.5
extrude "Extrude744" add sketch "mstand_26_457" along normal blind 6 from surface at 3 bodies 31
sketch "mpilot_26_457" plane through (0, 0, 0) normal (0, 0, 1) x (1, 0, 0)
  circle A0 centre (132.6, 65.7) radius 1.35
extrude "Extrude745" cut sketch "mpilot_26_457" against normal blind 7 from surface at 9 bodies 31
sketch "mstand_546_508" plane through (0, 0, 0) normal (0, 0, 1) x (1, 0, 0)
  circle A0 centre (184.6, 70.8) radius 3.5
extrude "Extrude746" add sketch "mstand_546_508" along normal blind 6 from surface at 3 bodies 31
sketch "mpilot_546_508" plane through (0, 0, 0) normal (0, 0, 1) x (1, 0, 0)
  circle A0 centre (184.6, 70.8) radius 1.35
extrude "Extrude747" cut sketch "mpilot_546_508" against normal blind 7 from surface at 9 bodies 31
sketch "mstand_533_25" plane through (0, 0, 0) normal (0, 0, 1) x (1, 0, 0)
  circle A0 centre (183.3, 22.5) radius 3.5
extrude "Extrude748" add sketch "mstand_533_25" along normal blind 6 from surface at 3 bodies 31
sketch "mpilot_533_25" plane through (0, 0, 0) normal (0, 0, 1) x (1, 0, 0)
  circle A0 centre (183.3, 22.5) radius 1.35
extrude "Extrude749" cut sketch "mpilot_533_25" against normal blind 7 from surface at 9 bodies 31
sketch "mstand_26_177" plane through (0, 0, 0) normal (0, 0, 1) x (1, 0, 0)
  circle A0 centre (132.6, 37.7) radius 3.5
extrude "Extrude750" add sketch "mstand_26_177" along normal blind 6 from surface at 3 bodies 31
sketch "mpilot_26_177" plane through (0, 0, 0) normal (0, 0, 1) x (1, 0, 0)
  circle A0 centre (132.6, 37.7) radius 1.35
extrude "Extrude751" cut sketch "mpilot_26_177" against normal blind 7 from surface at 9 bodies 31
sketch "rmnewboss_257_420" plane through (0, 0, 0) normal (0, 0, 1) x (1, 0, 0)
  circle A0 centre (25.7, 42) radius 4.5
extrude "Extrude752" cut sketch "rmnewboss_257_420" along normal blind 4.02 from surface at -44.01 bodies 3
sketch "rmnewboss_537_420" plane through (0, 0, 0) normal (0, 0, 1) x (1, 0, 0)
  circle A0 centre (53.7, 42) radius 4.5
extrude "Extrude753" cut sketch "rmnewboss_537_420" along normal blind 4.02 from surface at -44.01 bodies 3
sketch "rmnewboss_105_927" plane through (0, 0, 0) normal (0, 0, 1) x (1, 0, 0)
  circle A0 centre (10.5, 92.7) radius 4.5
extrude "Extrude754" cut sketch "rmnewboss_105_927" along normal blind 4.02 from surface at -44.01 bodies 3
sketch "rmnewboss_588_940" plane through (0, 0, 0) normal (0, 0, 1) x (1, 0, 0)
  circle A0 centre (58.8, 94) radius 4.5
extrude "Extrude755" cut sketch "rmnewboss_588_940" along normal blind 4.02 from surface at -44.01 bodies 3
move_body "Move4" bodies 31 to x (0, 1, 0) y (-1, 0, 0) z (0, 0, 1) at (144, -110, 0)
move_body "Move5" bodies 31 to x (1, 0, 0) y (0, 1, 0) z (0, 0, 1) at (-40, -10, 0)
move_body "Move6" bodies 31 to x (1, 0, 0) y (0, 1, 0) z (0, 0, 1) at (0, 0, -47)
combine "Combine1" operation add target body 3 tool bodies 31
extrude "Extrude756" add 1 faces at (103.4, 111.3333, -44) along direction (0, 0, -1) blind 30 on bodies 1 bodies 1
extrude "Extrude757" add 5 faces at (8.8283, 158.1943, -44) (89.6408, 119.1822, -44) (89.6408, 79.1822, -44) (14.951, 11.2913, -44) (96.451, 11.2913, -44) along direction (0, 0, -1) blind 30 on bodies 1 bodies 1
extrude "Extrude758" cut 1 faces at (103.4, 111.3333, -74) along direction (0, 0, 1) blind 30 on bodies 1 bodies 1
extrude "Extrude759" cut 5 faces at (14.951, 11.2913, -74) (96.451, 11.2913, -74) (89.6408, 79.1822, -74) (8.8283, 158.1943, -74) (89.6408, 119.1822, -74) along direction (0, 0, 1) blind 30 on bodies 1 bodies 1
extrude "Extrude760" add 1 faces at (42.2667, 76.8, -4.5333) along direction (0, 1, 0) blind 1 on bodies 1 bodies 1
extrude "Extrude761" cut 1 faces at (18.2, 96.9333, -5.0667) along direction (-1, 0, 0) blind 4 on bodies 1 bodies 1
extrude "Extrude762" add 1 faces at (5.3065, 19.9512, -9.4) along direction (0, 0, -1) blind 1 on bodies 1 bodies 1
extrude "Extrude763" add 1 faces at (77.2135, 69.6913, -9.4) along direction (0, 0, -1) blind 1 on bodies 1 bodies 1
extrude "Extrude764" add 1 faces at (94.2935, 54.1985, -9.4) along direction (0, 0, -1) blind 1 on bodies 1 bodies 1
extrude "Extrude765" add 1 faces at (56.1862, 13.8981, -9.4) along direction (0, 0, -1) blind 1 on bodies 1 bodies 1
sketch "Sketch652" plane through (0, 0, -5.6) normal (0, 0, 1) x (-1, 0, 0)
  line L0 (-78, -84.4) -> (-23.7, -84.4)
  line L1 (-23.7, -84.4) -> (-23.7, -127.6)
  line L2 (-23.7, -127.6) -> (-78, -127.6)
  line L3 (-78, -127.6) -> (-78, -84.4)
  line L4 (-14.2, -77.8) -> (-90.4, -77.8)
  line L5 (-90.4, -77.8) -> (-90.4, -135.2)
  line L6 (-90.4, -135.2) -> (-14.2, -135.2)
  line L7 (-14.2, -135.2) -> (-14.2, -77.8)
  line L8 (-14.2, -86.5718) -> (-25.1112, -77.8)
  dimension "d2223" = 14
  constraint coincident L7 L8.start
  constraint coincident L4 L8.end
  measures "d2223" distance of L8.start L8.end
extrude "Extrude766" add sketch "Sketch652" along normal blind 1.6 contours L4 L7 L8 bodies 1
sketch "Sketch653" plane through (0, 0, -4) normal (0, 0, 1) x (-1, 0, 0)
  circle A0 centre (-40, -69) radius 7.2
  line L0 (-15.4433, -75.9) -> (-19.5567, -75.9)
  arc A1 (-15.4433, -75.9) -> (-19.5567, -75.9) centre (-17.5, -69) ccw
  line L1 (-71.3, -25.8) -> (-59, -25.8)
  line L2 (-59, -25.8) -> (-59, -38.2)
  line L3 (-59, -38.2) -> (-71.3, -38.2)
  line L4 (-71.3, -38.2) -> (-71.3, -50.5)
  line L5 (-71.3, -50.5) -> (-83.7, -50.5)
  line L6 (-83.7, -50.5) -> (-83.7, -38.2)
  line L7 (-83.7, -38.2) -> (-96, -38.2)
  line L8 (-96, -38.2) -> (-96, -25.8)
  line L9 (-96, -25.8) -> (-83.7, -25.8)
  line L10 (-83.7, -25.8) -> (-83.7, -13.5)
  line L11 (-83.7, -13.5) -> (-71.3, -13.5)
  line L12 (-71.3, -13.5) -> (-71.3, -25.8)
  line L13 (-48.5, -21) -> (-11.5, -21)
  line L14 (-11.5, -21) -> (-11.5, -44)
  line L15 (-11.5, -44) -> (-48.5, -44)
  line L16 (-48.5, -44) -> (-48.5, -21)
  line L17 (-30.5, -51.1) -> (-30.5, -59.7)
  line L18 (-30.5, -59.7) -> (-45.5, -59.7)
  line L19 (-45.5, -59.7) -> (-45.5, -51.1)
  line L20 (-45.5, -51.1) -> (-30.5, -51.1)
  line L21 (-49.5, -51.1) -> (-49.5, -59.7)
  line L22 (-49.5, -59.7) -> (-64.5, -59.7)
  line L23 (-64.5, -59.7) -> (-64.5, -51.1)
  line L24 (-64.5, -51.1) -> (-49.5, -51.1)
  line L25 (-86, -64.5) -> (-99.5, -64.5)
  line L26 (-99.5, -64.5) -> (-99.5, -63)
  line L27 (-99.5, -63) -> (-86, -63)
  line L28 (-86, -63) -> (-86, -64.5)
  line L29 (-86, -67.5) -> (-99.5, -67.5)
  line L30 (-99.5, -67.5) -> (-99.5, -66)
  line L31 (-99.5, -66) -> (-86, -66)
  line L32 (-86, -66) -> (-86, -67.5)
  line L33 (-86, -73.5) -> (-99.5, -73.5)
  line L34 (-99.5, -73.5) -> (-99.5, -72)
  line L35 (-99.5, -72) -> (-86, -72)
  line L36 (-86, -72) -> (-86, -73.5)
  line L37 (-86, -70.5) -> (-99.5, -70.5)
  line L38 (-99.5, -70.5) -> (-99.5, -69)
  line L39 (-99.5, -69) -> (-86, -69)
  line L40 (-86, -69) -> (-86, -70.5)
  line L41 (-105, -43.7) -> (-105, -126.3)
  line L42 (-105, -126.3) -> (-103, -126.3)
  line L43 (-103, -126.3) -> (-103, -155.3758)
  arc A2 (-54, -141) -> (-103, -155.3758) centre (358, -1636) ccw
  arc A3 (0, -136) -> (-54, -141) centre (-11.7114, -303.6168) ccw
  line L44 (0, -136) -> (0, -6)
  arc A4 (0, -6) -> (-6, 0) centre (-6, -6) ccw
  line L45 (-6, 0) -> (-99, 0)
  arc A5 (-99, 0) -> (-104.6569, -4) centre (-99, -6) ccw
  line L46 (-104.6569, -4) -> (-103, -4)
  line L47 (-103, -4) -> (-103, -43.7)
  line L48 (-103, -43.7) -> (-105, -43.7)
  line L49 (-14.2, -135.2) -> (-90.4, -135.2)
  line L50 (-90.4, -135.2) -> (-90.4, -77.8)
  line L51 (-90.4, -77.8) -> (-25.1112, -77.8)
  line L52 (-25.1112, -77.8) -> (-14.2, -86.5718)
  line L53 (-14.2, -86.5718) -> (-14.2, -135.2)
  line L54 (-14.2, -135.2) -> (-90.4, -135.2)
  line L55 (-90.4, -135.2) -> (-90.4, -77.8)
  line L56 (-90.4, -77.8) -> (-25.1112, -77.8)
  line L57 (-14.2, -86.5718) -> (-14.2, -135.2)
  line L58 (-14.2, -86.5718) -> (-25.1112, -77.8)
  line L59 (-23.7, -127.6) -> (-78, -127.6)
  line L60 (-78, -127.6) -> (-78, -84.4)
  line L61 (-78, -84.4) -> (-23.7, -84.4)
  line L62 (-23.7, -84.4) -> (-23.7, -127.6)
  constraint perpendicular L54 L55
  constraint parallel L54 L56
  constraint parallel L55 L57
  constraint coincident L49.end L50.start
  constraint perpendicular L50 L54
  constraint coincident L49.start L53.end
  constraint coincident L52.end L53.start
  constraint coincident L51.end L52.start
  constraint perpendicular L59 L60
  constraint parallel L59 L61
  constraint parallel L60 L62
  constraint horizontal L59
extrude "Extrude767" add sketch "Sketch653" along normal blind 1 separate body contours L49 L50 L51 L52 L53 L54 L55 L56 L57 L58 makes body 32
sketch "Sketch654" plane through (0, 0, -3) normal (0, 0, 1) x (-1, 0, 0)
  line L0 (-78, -84.4) -> (-23.7, -84.4)
  line L1 (-23.7, -84.4) -> (-23.7, -127.6)
  line L2 (-23.7, -127.6) -> (-78, -127.6)
  line L3 (-78, -127.6) -> (-78, -84.4)
  line L4 (-14.2, -135.2) -> (-14.2, -86.5718)
  line L5 (-14.2, -86.5718) -> (-25.1112, -77.8)
  line L6 (-25.1112, -77.8) -> (-90.4, -77.8)
  line L7 (-90.4, -77.8) -> (-90.4, -135.2)
  line L8 (-90.4, -135.2) -> (-14.2, -135.2)
  circle A0 centre (-48, -131) radius 1
  circle A1 centre (-55, -131) radius 1
  circle A2 centre (-30, -81) radius 2.25
  dimension "d2228" = 2
  dimension "d2229" = 4.5
  measures "d2228" diameter of A1
  measures "d2229" diameter of A2
extrude "Extrude768" add sketch "Sketch654" along normal blind 0.4 contours A0 | A1 | A2 bodies 32
extrude "Extrude769" cut 1 faces at (27.5, 153.3333, 1.2) along direction (-1, 0, 0) blind 1.5 on bodies 1 bodies 1
extrude "Extrude770" cut 1 faces at (26, 156.6667, -3.5667) along direction (-1, 0, 0) blind 1 on bodies 1 bodies 1
extrude "Extrude771" cut 1 faces at (51.5, 0.8, -31.5) along direction (0, 0, -1) blind 4 on bodies 1 bodies 1
extrude "Extrude772" cut 1 faces at (45.5, 0.8, -33) along direction (-1, 0, 0) blind 2 on bodies 1 bodies 1
extrude "Extrude773" cut 1 faces at (54.5, 0.8, -30.5) along direction (1, 0, 0) blind 2 on bodies 1 bodies 1
sketch "dome2_plug" plane through (0, 0, 0) normal (0, 0, 1) x (1, 0, 0)
  circle A0 centre (19, 155) radius 10
extrude "Extrude774" add sketch "dome2_plug" along normal blind 2.2 from surface at 5.8 separate body makes body 33
ref_plane "WorkPlane68" through (0, 155, 0) normal (0, 1, 0) x (0, 0, 1)
sketch "dome2_prof" plane through (0, 155, 0) normal (0, 1, 0) x (1, 0, 0)
  arc A0 (19, -12) -> (29, -8) centre (19, 2.5) ccw
  line L0 (29, -8) -> (19, -8)
  line L1 (19, -8) -> (19, -12)
revolve "Revolve3" add sketch "dome2_prof" angle 360 about axis through (19, 155, 8) along (0, 0, 1) bodies 33
shell "Shell12" thickness 1.5 removed faces 1 at (22.0405, 153.0569, 5.8) on bodies 33
sketch "ring_flush" plane through (0, 0, 0) normal (0, 0, 1) x (1, 0, 0)
  circle A0 centre (19, 155) radius 13.3
  circle A1 centre (19, 155) radius 11.25
extrude "Extrude777" add sketch "ring_flush" along normal blind 2.2 from surface at 5.8 separate body makes body 34
sketch "dome_skirt" plane through (0, 0, 0) normal (0, 0, 1) x (1, 0, 0)
  circle A0 centre (19, 155) radius 11.15
  circle A1 centre (19, 155) radius 10
extrude "Extrude778" add sketch "dome_skirt" along normal blind 2.2 from surface at 5.8 bodies 33
extrude "Extrude779" add 1 faces at (29, 156.6667, 1.2) along direction (-1, 0, 0) blind 2 on bodies 1 bodies 1 33
extrude "Extrude780" cut 1 faces at (25, 156.6667, -3.5667) along direction (-1, 0, 0) blind 2 on bodies 1 bodies 1
extrude "Extrude781" add 1 faces at (27, 155.9574, -3.4) along direction (-1, 0, 0) blind 1 on bodies 1 bodies 1
extrude "Extrude782" cut 1 faces at (23, 156.6667, -3.5667) along direction (-1, 0, 0) blind 2 on bodies 1 bodies 1
extrude "Extrude783" add 1 faces at (21, 156.6667, -3.5667) along direction (1, 0, 0) blind 1 on bodies 1 bodies 1
sketch "remove_tub_dome" plane through (0, 0, 0) normal (0, 0, 1) x (1, 0, 0)
  circle A0 centre (19, 155) radius 13.6
extrude "Extrude785" cut sketch "remove_tub_dome" along normal blind 6 from surface at 8 bodies 1
sketch "clear_recess_dome" plane through (0, 0, 0) normal (0, 0, 1) x (1, 0, 0)
  circle A0 centre (19, 155) radius 13.3
extrude "Extrude786" cut sketch "clear_recess_dome" along normal blind 2.2 from surface at 5.8 bodies 1
move_body "Move7" bodies 32 to x (1, 0, 0) y (0, 1, 0) z (0, 0, 1) at (0, 0, -1.6)
sketch "bez_shrink" plane through (0, 0, 0) normal (0, 0, 1) x (1, 0, 0)
  line L0 (13.2, 76.8) -> (91.4, 76.8)
  line L1 (91.4, 76.8) -> (91.4, 136.2)
  line L2 (91.4, 136.2) -> (13.2, 136.2)
  line L3 (13.2, 136.2) -> (13.2, 76.8)
  line L4 (14.45, 78.05) -> (90.15, 78.05)
  line L5 (90.15, 78.05) -> (90.15, 134.95)
  line L6 (90.15, 134.95) -> (14.45, 134.95)
  line L7 (14.45, 134.95) -> (14.45, 78.05)
extrude "Extrude787" cut sketch "bez_shrink" along normal blind 3.4 from surface at -6.6 bodies 32
sketch "Sketch666" plane through (130, 0, 0) normal (1, 0, 0) x (0, 1, 0)
  line L0 (90.5, -5) -> (79.5, -5)
  line L1 (79.5, -5) -> (79.5, -9.6)
  line L2 (79.5, -9.6) -> (90.5, -9.6)
  line L3 (90.5, -9.6) -> (90.5, -5)
extrude "Extrude788" cut 1 faces at (130, 83.1667, -8.0665) along direction (-1, 0, 0) blind 2.5 on bodies 4 bodies 4 5
extrude "Extrude789" cut 1 faces at (129.3265, 79.5, -4.9047) along direction (0, 1, 0) blind 11 on bodies 4 bodies 4
sketch "Sketch667" plane through (130, 0, 0) normal (-1, 0, 0) x (0, -1, 0)
  line L0 (-90.5, -9) -> (-79.5, -9)
  line L1 (-79.5, -9) -> (-79.5, -7)
  line L2 (-79.5, -7) -> (-90.5, -7)
  line L3 (-90.5, -7) -> (-90.5, -9)
extrude "Extrude790" add 1 faces at (130, 83.1667, -8.3333) along direction (-1, 0, 0) blind 2.1 on bodies 5 bodies 5
extrude "Extrude791" cut 1 faces at (127.5, 83.1667, -8.0667) along direction (-1, 0, 0) blind 0.1 on bodies 4 bodies 4
extrude "Extrude792" cut 1 faces at (128, 86.8333, -1.6665) along direction (-1, 0, 0) blind 0.1 on bodies 4 bodies 4
extrude "Extrude793" cut 1 faces at (127.9, 86.8333, -1.6665) along direction (-1, 0, 0) blind 0.1 on bodies 4 bodies 4
extrude "Extrude794" cut 1 faces at (127.8, 86.8333, -1.6665) along direction (-1, 0, 0) blind 0.3 on bodies 4 bodies 4
sketch "Sketch668" plane through (127.5, 0, 0) normal (1, 0, 0) x (0, 1, 0)
  line L0 (44, -5) -> (126, -5)
  line L1 (126, -5) -> (126, 0)
  line L2 (126, 0) -> (44, 0)
  line L3 (44, 0) -> (44, -5)
ref_plane "WorkPlane69" through (0, 0, 0) normal (0, 0, 1) x (1, 0, 0)
ref_plane "WorkPlane70" through (0, 0, -2.4) normal (0, 0, 1) x (1, 0, 0)
ref_plane "WorkPlane71" through (0, 0, 0) normal (0, 0, 1) x (1, 0, 0)
ref_plane "WorkPlane72" through (0, 0, -2.4) normal (0, 0, 1) x (1, 0, 0)
sketch "rc_disc_Cap_Back" plane through (0, 0, 0) normal (0, 0, 1) x (1, 0, 0)
  circle A0 centre (40, 69) radius 7
extrude "Extrude811" add sketch "rc_disc_Cap_Back" along normal blind 2 separate body makes body 35
ref_plane "WorkPlane73" through (0, 0, 0) normal (0, 0, 1) x (1, 0, 0)
ref_plane "WorkPlane74" through (0, 0, -2.4) normal (0, 0, 1) x (1, 0, 0)
sketch "rc_st_Cap_Back" plane through (0, 0, 0) normal (0, 0, 1) x (1, 0, 0)
  circle A0 centre (40, 69) radius 7.1
sketch "rc_sb_Cap_Back" plane through (0, 0, -2.4) normal (0, 0, 1) x (1, 0, 0)
  circle A0 centre (40, 69) radius 6.6
loft "Loft3" add profiles "rc_st_Cap_Back", "rc_sb_Cap_Back" section 1 section 2 bodies 35
sketch "rc_sk_Cap_Back" plane through (0, 0, 0) normal (0, 0, 1) x (1, 0, 0)
  circle A0 centre (40, 69) radius 2.5
extrude "Extrude812" cut sketch "rc_sk_Cap_Back" along normal blind 1 from surface at -2.4 bodies 35
fillet "Fillet53" radius 1.5 1 edges at (33.4737, 66.4687, 2) on bodies 35
sketch "rc_disc_Cap_btn9" plane through (0, 0, 0) normal (0, 0, 1) x (1, 0, 0)
  circle A0 centre (30, 32.5) radius 7
extrude "Extrude813" add sketch "rc_disc_Cap_btn9" along normal blind 2 separate body makes body 36
ref_plane "WorkPlane75" through (0, 0, 0) normal (0, 0, 1) x (1, 0, 0)
ref_plane "WorkPlane76" through (0, 0, -2.4) normal (0, 0, 1) x (1, 0, 0)
sketch "rc_st_Cap_btn9" plane through (0, 0, 0) normal (0, 0, 1) x (1, 0, 0)
  circle A0 centre (30, 32.5) radius 7.1
sketch "rc_sb_Cap_btn9" plane through (0, 0, -2.4) normal (0, 0, 1) x (1, 0, 0)
  circle A0 centre (30, 32.5) radius 6.6
loft "Loft4" add profiles "rc_st_Cap_btn9", "rc_sb_Cap_btn9" section 1 section 2 bodies 36
sketch "rc_sk_Cap_btn9" plane through (0, 0, 0) normal (0, 0, 1) x (1, 0, 0)
  circle A0 centre (30, 32.5) radius 2.5
extrude "Extrude814" cut sketch "rc_sk_Cap_btn9" along normal blind 1 from surface at -2.4 bodies 36
fillet "Fillet54" radius 1.5 1 edges at (23.4737, 29.9687, 2) on bodies 36
sketch "rc_disc_Cap_Select" plane through (0, 0, 0) normal (0, 0, 1) x (1, 0, 0)
  circle A0 centre (17.5, 69) radius 7
extrude "Extrude815" add sketch "rc_disc_Cap_Select" along normal blind 2 separate body makes body 37
ref_plane "WorkPlane77" through (0, 0, 0) normal (0, 0, 1) x (1, 0, 0)
ref_plane "WorkPlane78" through (0, 0, -2.4) normal (0, 0, 1) x (1, 0, 0)
sketch "rc_st_Cap_Select" plane through (0, 0, 0) normal (0, 0, 1) x (1, 0, 0)
  circle A0 centre (17.5, 69) radius 7.1
sketch "rc_sb_Cap_Select" plane through (0, 0, -2.4) normal (0, 0, 1) x (1, 0, 0)
  circle A0 centre (17.5, 69) radius 6.6
loft "Loft5" add profiles "rc_st_Cap_Select", "rc_sb_Cap_Select" section 1 section 2 bodies 37
sketch "rc_sk_Cap_Select" plane through (0, 0, 0) normal (0, 0, 1) x (1, 0, 0)
  circle A0 centre (17.5, 69) radius 2.5